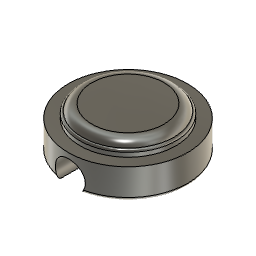
BeerStand (Autodesk Fusion 360 design; units mm, degrees)
Autodesk Fusion 360 part; units mm, degrees
note: some values were not read from the file. Chosen so that the rebuilt part matches the saved one: which face or edge a step refers to.
sketch "Sketch1" plane through (0, 0, 0) normal (0, 0, 1) x (1, 0, 0)
  circle A0 centre (0, 0) radius 22.5
  dimension "d1" = 45
  constraint coincident A0.centre origin
  measures "d1" diameter of A0
extrude "Extrude1" add sketch "Sketch1" along normal blind 2
fillet "Fillet1" radius 1 1 faces at (2.0784, -12.7768, 2)
sketch "Sketch2" plane through (0, 0, 2) normal (0, 0, 1) x (-1, 0, 0)
  circle A0 centre (0, 0) radius 21.5
  circle A1 centre (0, 0) radius 21.5
  constraint concentric A0 A1
extrude "Extrude2" add sketch "Sketch2" along normal blind 3
fillet "Fillet2" radius 5 1 faces at (0.08, -1.0681, 5)
extrude "Extrude3" add 1 faces at (2.0784, -12.7768, 0) along direction (0, 0, -1) blind 1
move_face "MoveFace1" to x (1, 0, 0) y (0, 1, 0) z (0, 0, 1) at (0, 0, 1) 5 faces at (22.472, -1.1215, 0.6667) (21.2918, 2.1306, 2.2189) (15.6977, -16.0941, 1.1893) (3.5656, 9.0849, 5) (2.0784, -12.7768, -1)
sketch "Sketch3" plane through (0, 0, 0) normal (0, 0, 1) x (1, 0, 0)
  circle A0 centre (0, 0) radius 28
  dimension "d12" = 56
  constraint coincident A0.centre origin
  measures "d12" diameter of A0
extrude "Extrude4" add sketch "Sketch3" against normal blind 14
sketch "Sketch4" plane through (0, 0, 0) normal (0, 1, 0) x (1, 0, 0)
  circle A0 centre (0.0496, 9.4822) radius 7
  dimension "d15" = 14
  measures "d15" diameter of A0
extrude "Extrude5" cut sketch "Sketch4" along normal mid plane 198
fillet "Fillet3" radius 1.5 3 edges at (21.6229, -17.789, -14) (-28, 0, -14) (21.6229, 17.789, -14)
move_body "Move1" bodies 1 to x (1, 0, 0) y (0, 1, 0) z (0, 0, 1) at (0, 0, 14)
